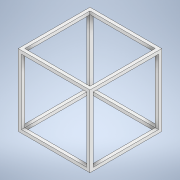
# Autodesk Inventor part: Hollow_Cube
Saved by Autodesk Inventor 2020 (Build 240168000, 168)
## iProperties
Created: 2021-12-16
Part Number: Hollow_Cube
Material: ABS Plastic
Document SubType Name: Modeling
Designer: Umur Batuhan Özmen
Density: 1.06 g/cm^3
Appearance: Smooth - White
Author: Umur Batuhan Özmen
## iProperties of the stored document _3DPrint.ipt
Created: 2021-12-16
Part Number: _3DPrint
Material: Generic
Document SubType Name: Modeling
Designer: Umur Batuhan Özmen
Density: 1 g/cm^3
Appearance: Default
Author: Umur Batuhan Özmen
Autodesk Inventor part; units mm, degrees
ref_plane "YZ Plane" through (0, 0, 0) normal (1, 0, 0) x (0, 1, 0)
ref_plane "XZ Plane" through (0, 0, 0) normal (0, 1, 0) x (-1, 0, 0)
ref_plane "XY Plane" through (0, 0, 0) normal (0, 0, 1) x (1, 0, 0)
sketch "Sketch1" plane through (0, 0, 0) normal (0, 1, 0) x (-1, 0, 0)
  line L0 (50, 50) -> (-50, 50)
  line L1 (-50, 50) -> (-50, -50)
  line L2 (-50, -50) -> (50, -50)
  line L3 (50, -50) -> (50, 50)
  line L4 (50, 50) -> (-50, -50) construction
  line L5 (-50, 50) -> (50, -50) construction
  line L6 (55, 55) -> (-55, 55)
  line L7 (-55, 55) -> (-55, -55)
  line L8 (-55, -55) -> (55, -55)
  line L9 (55, -55) -> (55, 55)
  line L10 (55, 55) -> (-55, -55) construction
  line L11 (-55, 55) -> (55, -55) construction
  point P0 (0, 0)
  dimension "d0" = 100
  dimension "d1" = 100
  dimension "d2" = 110
  dimension "d3" = 110
  constraints: 24 end point, 4 midpoint, 4 parallel, 2 horizontal, 2 perpendicular
  measures "d0" distance of L2.end L1.end
  measures "d1" distance of L1.end L0.end
  measures "d2" distance of L8.end L7.end
  measures "d3" distance of L7.end L6.end
extrude "Extrusion1" add sketch "Sketch1" against normal blind 110 contours L3 L2 L1 L0 | L9 L8 L7 L6
extrude "Extrusion2" cut sketch "Sketch1" against normal blind 110 contours L3 L2 L1 L0
sketch "Sketch2" plane through (-55, 0, 55) normal (0, 0, 1) x (1, 0, 0)
  line L0 (0, 0) -> (110, 0) projected
  line L1 (0, 0) -> (0, -110) projected
  line L2 (110, -110) -> (0, -110) projected
  line L3 (110, 0) -> (110, -110) projected
  line L4 (5, -5) -> (105, -5)
  line L5 (105, -5) -> (105, -105)
  line L6 (105, -105) -> (5, -105)
  line L7 (5, -105) -> (5, -5)
  line L8 (5, -5) -> (105, -105) construction
  line L9 (105, -5) -> (5, -105) construction
  point P0 (55, 0)
  point P1 (55, -55)
  dimension "d8" = 100
  dimension "d9" = 100
  constraints: 12 end point, 2 midpoint, 2 parallel, 1 horizontal, 1 perpendicular
  measures "d8" distance of L5.end L6.end
  measures "d9" distance of L4.end L5.end
extrude "Extrusion3" cut sketch "Sketch2" against normal blind 110 contours L4 L5 L6 L7
sketch "Sketch3" plane through (55, 0, 55) normal (1, 0, 0) x (0, 0, -1)
  line L0 (0, 0) -> (110, 0) projected
  line L1 (0, 0) -> (0, -110) projected
  line L2 (110, -110) -> (0, -110) projected
  line L3 (110, 0) -> (110, -110) projected
  line L4 (5, -5) -> (105, -5)
  line L5 (105, -5) -> (105, -105)
  line L6 (105, -105) -> (5, -105)
  line L7 (5, -105) -> (5, -5)
  line L8 (5, -5) -> (105, -105) construction
  line L9 (105, -5) -> (5, -105) construction
  point P0 (55, 0)
  point P1 (55, -55)
  dimension "d12" = 100
  dimension "d13" = 100
  constraints: 12 end point, 2 midpoint, 2 parallel, 1 horizontal, 1 perpendicular
  measures "d12" distance of L5.end L6.end
  measures "d13" distance of L4.end L5.end
extrude "Extrusion4" cut sketch "Sketch3" against normal blind 110 contours L4 L5 L6 L7
body "Solid1"
